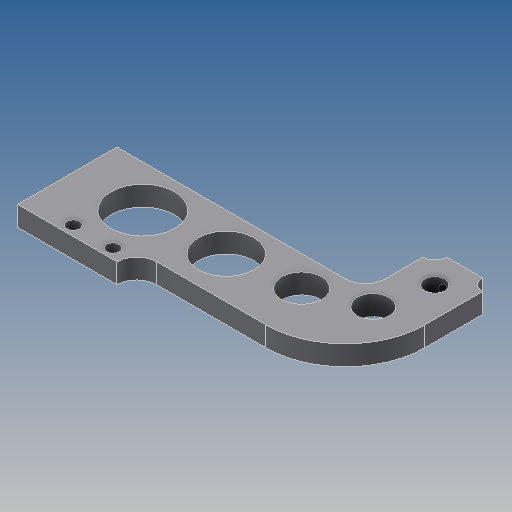
# Autodesk Inventor part: Lagerarm
Saved by Autodesk Inventor 2018 (Build 220112000, 112)
## iProperties
Created: 2018-09-11
Part Number: Lagerarm
Material: Generisch
Document SubType Name: Modeling
Designer: M.Knabel
Density: 1 g/cm^3
Appearance: Vorgabe
Mass: 6.58509 g
Surface Area: 47.9829 cm^2
Volume: 6.58509 cm^3
Author: M.Knabel
Autodesk Inventor part; units mm, degrees
note: some values were not read from the file. Chosen so that the rebuilt part matches the saved one: direction of "Bohrung2".
ref_plane "YZ Plane" through (0, 0, 0) normal (1, 0, 0) x (0, 1, 0)
ref_plane "XZ Plane" through (0, 0, 0) normal (0, 1, 0) x (-1, 0, 0)
ref_plane "XY Plane" through (0, 0, 0) normal (0, 0, 1) x (1, 0, 0)
sketch "Skizze1" plane through (0, 0, 0) normal (0, 0, 1) x (1, 0, 0)
  line L0 (-16.3284, 0) -> (97.9706, 0) projected
  line L1 (0, -8.5) -> (0, 51) projected
  line L2 (0, 0) -> (0, 25)
  line L3 (0, 25) -> (57.5, 25)
  line L4 (62.5, 30) -> (62.5, 39.5)
  line L5 (77.5, 39.5) -> (77.5, 25)
  line L6 (57.5, 5) -> (30, 5)
  line L7 (25, 0) -> (25, 0)
  arc A0 (57.5, 5) -> (77.5, 25) centre (57.5, 25) ccw
  arc A1 (57.5, 25) -> (62.5, 30) centre (57.5, 30) ccw
  arc A2 (30, 5) -> (25, 0) centre (30, 0) ccw
  arc A3 (62.5, 39.5) -> (65.5, 42.5) centre (62.5, 42.5) ccw
  arc A4 (74.5, 42.5) -> (77.5, 39.5) centre (77.5, 42.5) ccw
  line L8 (65.5, 42.5) -> (74.5, 42.5)
  point P0 (62.5, 25)
  point P1 (77.5, 5)
  point P2 (25, 5)
  dimension "d0" = 77.5
  dimension "d3" = 25
  dimension "d4" = 5
  dimension "d5" = 25
  dimension "d11" = 20
  dimension "d12" = 5
  dimension "d19" = 15
  dimension "d21" = 42.5
  dimension "d22" = 3
  dimension "d23" = 3
  constraints: 14 end point, 12 point on line, 10 point on circle, 6 tangent, 5 centre point, 2 horizontal, 2 perpendicular, 1 equal radius, 1 vertical
  measures "d0" distance between parallel lines of L5 L1
  measures "d3" distance between parallel lines of L0 L3
  measures "d4" distance between parallel lines of L0 L6
  measures "d5" distance between parallel lines of L1 L7
  measures "d11" radius of A0
  measures "d12" radius of A1
  measures "d19" distance between parallel lines of L5 L4
  measures "d21" distance between parallel lines of L0 L8
  measures "d22" radius of A3
  measures "d23" radius of A4
extrude "Grundkörper" add sketch "Skizze1" along normal blind 5
sketch "Skizze2" plane through (0, 0, 5) normal (0, 0, 1) x (1, 0, 0)
  line L0 (0, -8.5) -> (0, 51) projected
  line L1 (-15.5, 0) -> (93, 0) projected
  line L2 (30, 5) -> (57.5, 5) projected
  circle A0 centre (11.5, 2.5) radius 1.6
  circle A1 centre (17, 14.5) radius 8
  circle A2 centre (21.5, 2.5) radius 1.6
  circle A3 centre (37, 15.5) radius 7
  circle A4 centre (54, 17.5) radius 5
  circle A5 centre (67, 22.5) radius 4
  circle A6 centre (70, 35) radius 2.5
  point P0 (0, 0)
  dimension "d24" = 11.5
  dimension "d25" = 10
  dimension "d26" = 2.5
  dimension "d27" = 2.5
  dimension "d28" = 14.5
  dimension "d29" = 17
  dimension "d30" = 10.5
  dimension "d31" = 37
  dimension "d32" = 12.5
  dimension "d33" = 54
  dimension "d34" = 17.5
  dimension "d35" = 67
  dimension "d36" = 70
  dimension "d37" = 35
  dimension "d38" = 16
  dimension "d39" = 3.2
  dimension "d40" = 3.2
  dimension "d41" = 14
  dimension "d42" = 10
  dimension "d43" = 8
  dimension "d44" = 5
  constraints: 7 centre point, 7 coincident
  measures "d24" distance from line of L0 point (11.5, 2.5)
  measures "d25" distance of point (21.5, 2.5) point (11.5, 2.5)
  measures "d26" distance from line of L1 point (11.5, 2.5)
  measures "d27" distance from line of L1 point (21.5, 2.5)
  measures "d28" distance from line of L1 point (17, 14.5)
  measures "d29" distance from line of L0 point (17, 14.5)
  measures "d30" distance from line of point (37, 15.5) L2
  measures "d31" distance from line of point (37, 15.5) L0
  measures "d32" distance from line of L2 point (54, 17.5)
  measures "d33" distance from line of point (54, 17.5) L0
  measures "d34" distance from line of point (67, 22.5) L2
  measures "d35" distance from line of point (67, 22.5) L0
  measures "d36" distance from line of point (70, 35) L0
  measures "d37" distance from line of L1 point (70, 35)
  measures "d38" diameter of A1
  measures "d39" diameter of A0
  measures "d40" diameter of A2
  measures "d41" diameter of A3
  measures "d42" diameter of A4
  measures "d43" diameter of A5
  measures "d44" diameter of A6
extrude "Extrusion2" cut sketch "Skizze2" against normal through all
sketch "Skizze3" plane through (0, 0, 0) normal (-1, 0, 0) x (0, 0, 1)
  line L0 (0, -8.5) -> (0, 51) projected
  line L1 (-1, 0) -> (6, 0) projected
  point P0 (0, 0)
  point P1 (2.5, 10)
  dimension "d47" = 10
  dimension "d48" = 2.5
  measures "d47" distance from line of L1 point (2.5, 10)
  measures "d48" distance from line of L0 point (2.5, 10)
hole "Bohrung1" at (0, 10, 2.5) direction (1, 0, 0) diameter 2.459 depth 7 tip angle 118 thread size "M3x0.5" class "6H" standard "ISO Metric profile"
sketch "Skizze4" plane through (65.5, 42.5, 0) normal (0, 1, 0) x (1, 0, 0)
  line L0 (-81, 0) -> (27.5, 0) projected
  line L1 (12, 0) -> (12, -5) projected
  point P0 (-65.5, 0)
  point P1 (4.5, -2.5)
  dimension "d56" = 7.5
  dimension "d57" = 2.5
  measures "d56" distance from line of point (4.5, -2.5) L1
  measures "d57" distance from line of L0 point (4.5, -2.5)
hole "Bohrung2" at (70, 42.5, 2.5) direction (0, -1, 0) diameter 2.459 end up to surface thread size "M3x0.5" class "6H" standard "ISO Metric profile"
